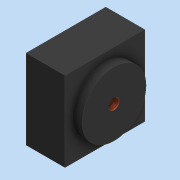
# Autodesk Inventor part: 카메라
Saved by Autodesk Inventor 2020 (Build 240168000, 168)
## iProperties
Created: 2020-05-05
Part Number: 카메라
Material: 일반
Document SubType Name: Modeling
Designer: sbahn
Density: 1 g/cm^3
Appearance: 고무 - 검은색
Author: sbahn
Autodesk Inventor part; units mm, degrees
ref_plane "YZ Plane" through (0, 0, 0) normal (1, 0, 0) x (0, 1, 0)
ref_plane "XZ Plane" through (0, 0, 0) normal (0, 1, 0) x (-1, 0, 0)
ref_plane "XY Plane" through (0, 0, 0) normal (0, 0, 1) x (1, 0, 0)
sketch "스케치1" plane through (0, 0, 0) normal (1, 0, 0) x (0, 1, 0)
  line L0 (4.3, 4.3) -> (-4.3, 4.3)
  line L1 (-4.3, 4.3) -> (-4.3, -4.3)
  line L2 (-4.3, -4.3) -> (4.3, -4.3)
  line L3 (4.3, -4.3) -> (4.3, 4.3)
  line L4 (4.3, 4.3) -> (-4.3, -4.3) construction
  line L5 (-4.3, 4.3) -> (4.3, -4.3) construction
  point P0 (0, 0)
  dimension "d0" = 8.6
  dimension "d1" = 8.6
  constraints: 12 end point, 2 midpoint, 2 parallel, 1 horizontal, 1 perpendicular
  measures "d0" distance of L2.end L1.end
  measures "d1" distance of L1.end L0.end
extrude "돌출1" add sketch "스케치1" along normal blind 4.2
sketch "스케치2" plane through (4.2, 0, 0) normal (1, 0, 0) x (0, 0, -1)
  circle A0 centre (0, 0) radius 3.45
  dimension "d4" = 6.9
  constraints: 1 centre point, 1 coincident
  measures "d4" diameter of A0
extrude "돌출2" add sketch "스케치2" along normal blind 1
sketch "스케치3" plane through (5.2, 0, 0) normal (1, 0, 0) x (0, 0, -1)
  circle A0 centre (0, 0) radius 0.5
  dimension "d7" = 1
  constraints: 1 centre point, 1 coincident
  measures "d7" diameter of A0
extrude "돌출3" cut sketch "스케치3" against normal blind 0.5
chamfer "모따기1" distance 0.1 angle 45 1 edges at (5.2, 0, 0.5)
